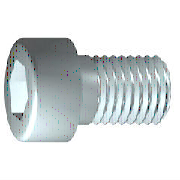
# Autodesk Inventor part: BS EN ISO 4762 - M3 x 10
Saved by Autodesk Inventor 2025.1 (Build 291241000, 241)
## iProperties
Created: 2024-01-20
Part Number: BS EN ISO 4762 - M3 x 10
Material: Acier, doux
Description: Vis cylindrique à six pans creux
Document SubType Name: Modeling
Standard: BS EN ISO 4762
Designer: felix
Standard Revision: 2004
Standards Organization: BSI
Language: fr-FR
Size Designation: M3 x 10
Categories: <MemberInstance><Categories><Category DisplayName="Visserie" InternalName="e4da775c-781d-43d5-af7c-5136215cf5a6" Mnemonic="FSTN"><Category DisplayName="Vis" InternalName="536e6df0-f778-49ac-b2f2-25c71d2aa0b2" Mnemonic="SCRW"><CategoryParameter DisplayName="Désignation du diamètre nominal" InternalName="03caf894-eafd-4c09-a035-916ac084b87b" Mnemonic="nomdiadesig"/><CategoryParameter DisplayName="Longueur nominale" InternalName="238ecbaf-3e6c-45dd-aa95-4068c8e0fd02" Mnemonic="nomlen"/><CategoryParameter DisplayName="Désignation du filetage" InternalName="586d5e89-370a-4089-914f-0110033585c7" Mnemonic="thrdesign"/><CategoryParameter DisplayName="Désignation de série de filetage" InternalName="87c5849c-b3a5-4c3e-9c9b-2feecef9be86" Mnemonic="thrserdsgn"/><CategoryParameter DisplayName="Diamètre nominal" InternalName="8bbe3f8e-44cf-40a9-a251-3a6edc8168d6" Mnemonic="nomdia"/><CategoryParameter DisplayName="Type de taraudage" InternalName="b4bbb7bc-d6aa-4c9f-a9a9-4152b9f6fe49" Mnemonic="thrtype"/><CategoryParameter DisplayName="Pas de filetage" InternalName="bb82302e-82d8-4176-8fc1-c5d7bb17d5ad" Mnemonic="pitch1"/><CategoryParameter DisplayName="Filets par unité" InternalName="bdc6e7d2-ffd0-4d9c-a173-16b95ebb912d" Mnemonic="thrperunit1"/><CategoryParameter DisplayName="Classe de filetage" InternalName="ebc0d23b-2cc6-4d2a-b376-d52aae53bab6" Mnemonic="thrclss"/><Category DisplayName="Tête creuse" InternalName="55e06bf3-7e58-486c-bbdc-745fcc60664d" Mnemonic="CLSCRW"><CategoryParameter DisplayName="Diamètre de tige" InternalName="179dbae3-102f-48bb-85fe-1e3ecd34f7cc" Mnemonic="grpdia"/><CategoryParameter DisplayName="Longueur de filetage" InternalName="3268731d-5f9a-4750-8b01-4a959c46fbf2" Mnemonic="thrlen"/><CategoryParameter DisplayName="Diamètre de tête" InternalName="46177176-dbdd-4a1b-aefd-4c60c45016af" Mnemonic="headdia"/><CategoryParameter DisplayName="Longueur de serrage" InternalName="52eab69f-422f-4795-9995-175a1b827e67" Mnemonic="grplen"/><CategoryParameter DisplayName="Type" InternalName="59a7e495-7a0c-4a5c-bdfd-c090c5f6e2db" Mnemonic="type"/><CategoryParameter DisplayName="Hauteur de tête" InternalName="99c92c4c-4a02-4ebe-9e64-948fb169e19e" Mnemonic="headh"/></Category></Category></Category><Category DisplayName="Type de données" InternalName="23b78d0f-2648-40c6-8793-ca6db495c9e8" Mnemonic="DATATYPE"><CategoryParameter DisplayName="AfficherNom" InternalName="05415f3d-3907-474b-a020-eb9d644f4cf3" Mnemonic="DISPLAYNAME"/><CategoryParameter DisplayName="Norme" InternalName="0c0a119c-1e12-4c84-803f-101930972f5e" Mnemonic="STANDARD"/><CategoryParameter DisplayName="Description" InternalName="13903e3d-64b1-4950-80da-f627842ea37f" Mnemonic="DESCRIPTION"/><CategoryParameter DisplayName="Désignation" InternalName="2675968c-4ce5-49e0-a4f5-552d29089031" Mnemonic="DESIGNATION"/><CategoryParameter DisplayName="Ligne par défaut" InternalName="2af9ec52-faaa-4026-b378-f9fa4afca842" Mnemonic="DEFAULTROW"/><CategoryParameter DisplayName="Nom de dossier" InternalName="3f06958e-8713-4116-9be7-ed6184ecc97b" Mnemonic="FOLDERNAME"/><CategoryParameter DisplayName="Guide révision" InternalName="45a75005-10b1-4dfc-8d6d-dfe629f0b93c" Mnemonic="REVISIONGUID"/><CategoryParameter DisplayName="NomFichier" InternalName="8b46a4cc-9585-4fed-90c3-899f57e09a73" Mnemonic="FILENAME"/><CategoryParameter DisplayName="OrgNorm" InternalName="8f5914e1-4693-403f-8ab5-d37768198c9d" Mnemonic="STDSORG"/><CategoryParameter DisplayName="Version de la famille" InternalName="914462f6-6e19-4b14-ba84-155b9680b1d0" Mnemonic="FAMILYREVISION"/><CategoryParameter DisplayName="Version standard" InternalName="91d5a463-65c2-4fde-b823-3b7fea5e8e17" Mnemonic="STANDARDREVISION"/><CategoryParameter DisplayName="Révision de membre" InternalName="a65d44b9-392f-4f4f-857b-e4b3d54996fe" Mnemonic="MEMBERREVISION"/><CategoryParameter DisplayName="DélimiterFormat" InternalName="bc51e27b-3422-4e78-93ef-cec197ddf230" Mnemonic="CLIPFORMAT"/><CategoryParameter DisplayName="Fabricant" InternalName="cd6c7a72-a28a-4e50-99a9-2c7f4e13e5ad" Mnemonic="MANUFACTURER"/><CategoryParameter DisplayName="NomInterne" InternalName="cf1d0246-76d9-4b4a-8305-fa0409afb5c1" Mnemonic="INTERNALNAME"/><CategoryParameter DisplayName="Métrique" InternalName="e2385c5b-1ea4-4823-96a8-8de651266ec3" Mnemonic="ISMETRIC"/><Category DisplayName="Pièce" InternalName="c0e0b642-3bcb-4cc8-9e80-f96d35c4afa4" Mnemonic="PART"><CategoryParameter DisplayName="Numéro de pièce" InternalName="016b6077-bfbe-49bd-92c9-d8d59c39c941" Mnemonic="PARTNUMBER"/><CategoryParameter DisplayName="Numéro de stock" InternalName="4dba7c1c-e26c-444e-836c-b08b433409a8" Mnemonic="STOCKNUMBER"/><CategoryParameter DisplayName="Clé matière" InternalName="5c9a8adb-dd2b-4535-b97f-0a94a95fe41f" Mnemonic="MATERIALKEY"/><CategoryParameter DisplayName="Matière" InternalName="818a152a-d3c3-49ca-80ee-df7d91421b8e" Mnemonic="MATERIAL"/></Category></Category><Category DisplayName="CarteHéritée" InternalName="cd87c42b-3e48-431e-b5c0-1cbeb14dfe77" Mnemonic="LEGACYMAP"><CategoryParameter DisplayName="ID membre DA unique" InternalName="0918ad47-427f-4fed-ae26-24c81c58f590" Mnemonic="DACOOKIE"/><CategoryParameter DisplayName="ID de fusion11" InternalName="0ee8fb18-e2ed-4f39-96f6-1f4b5f50aa71" Mnemonic="MERGE11"/><CategoryParameter DisplayName="ID membre CC unique" InternalName="5193edd4-b2b0-4ab4-9d54-de900eee34e0" Mnemonic="CCCOOKIE"/><CategoryParameter DisplayName="ID de division" InternalName="72b5c83c-be7f-45c4-ae51-9160ea6deb26" Mnemonic="SPLIT"/><CategoryParameter DisplayName="IDMembre" InternalName="8e5e0294-fc51-4c8f-b3d7-003dc5ed94f6" Mnemonic="MEMBERID"/><CategoryParameter DisplayName="NomCatologue" InternalName="d99d1e27-aa94-4de2-af4c-c348882a6f4f" Mnemonic="CATALOGNAME"/><CategoryParameter DisplayName="NuméroFamille" InternalName="e705e1f4-09cb-413e-91f9-551b4188271e" Mnemonic="FAMILYNUMBER"/></Category></Categories><FamilyTemplate Id="si0145"><FamilyTemplateParameters><FamilyTemplateParameter ObjectType="kUserParameterObject" ValueType="xs:double" Id="1" ObjectReferenceKey="GUL"/><FamilyTemplateParameter ObjectType="kUserParameterObject" ValueType="xs:double" Id="2" ObjectReferenceKey="SPD"/><FamilyTemplateParameter ObjectType="kUserParameterObject" ValueType="xs:double" Id="3" ObjectReferenceKey="NLG"/><FamilyTemplateParameter ObjectType="kUserParameterObject" ValueType="xs:double" Id="4" ObjectReferenceKey="KOD"/><FamilyTemplateParameter ObjectType="kUserParameterObject" ValueType="xs:double" Id="5" ObjectReferenceKey="TOA"/><FamilyTemplateParameter ObjectType="kUserParameterObject" ValueType="xs:double" Id="6" ObjectReferenceKey="GD1"/><FamilyTemplateParameter ObjectType="kUserParameterObject" ValueType="xs:double" Id="7" ObjectReferenceKey="GEL"/><FamilyTemplateParameter ObjectType="kUserParameterObject" ValueType="xs:double" Id="8" ObjectReferenceKey="SW"/><FamilyTemplateParameter ObjectType="kUserParameterObject" ValueType="xs:double" Id="9" ObjectReferenceKey="THREADDIA"/><FamilyTemplateParameter ObjectType="kUserParameterObject" ValueType="xs:double" Id="10" ObjectReferenceKey="INTI"/><FamilyTemplateParameter ObjectType="kUserParameterObject" ValueType="xs:double" Id="11" ObjectReferenceKey="BDM"/><FamilyTemplateParameter ObjectType="kUserParameterObject" ValueType="xs:double" Id="12" ObjectReferenceKey="FAWI"/><FamilyTemplateParameter ObjectType="kUserParameterObject" ValueType="xs:double" Id="13" ObjectReferenceKey="RR"/><FamilyTemplateParameter ObjectType="kUserParameterObject" ValueType="xs:double" Id="14" ObjectReferenceKey="KOH"/><FamilyTemplateParameter ObjectType="kUserParameterObject" ValueType="xs:double" Id="15" ObjectReferenceKey="TPU"/><FamilyTemplateParameter ObjectType="kUserParameterObject" ValueType="xs:double" Id="16" ObjectReferenceKey="PTC"/><FamilyTemplateParameter ObjectType="kUserParameterObject" ValueType="xs:double" Id="17" ObjectReferenceKey="NND"/><FamilyTemplateParameter ObjectType="kUserParameterObject" ValueType="xs:double" Id="18" ObjectReferenceKey="GD"/><FamilyTemplateParameter ObjectType="kUserParameterObject" ValueType="xs:double" Id="19" ObjectReferenceKey="GAL"/><FamilyTemplateParameter ObjectType="kUserParameterObject" ValueType="xs:double" Id="20" ObjectReferenceKey="E0"/><FamilyTemplateParameter ObjectType="kPropertyObject" ValueType="xs:string" Id="100" ObjectReferenceKey="{32853F0F-3444-11d1-9E93-0060B03C1CA6}" SubObjectId="52"/><FamilyTemplateParameter ObjectType="kPropertyObject" ValueType="xs:string" Id="105" ObjectReferenceKey="{32853F0F-3444-11d1-9E93-0060B03C1CA6}" SubObjectId="5"/><FamilyTemplateParameter ObjectType="kPartComponentDefinitionObject" ValueType="xs:string" Id="110" SubObjectId="Material"/><FamilyTemplateParameter ObjectType="kThreadFeatureObject" ValueType="xs:structure" Id="300" ObjectReferenceKey="1002000010000000a2070000000000008000000000000000" SubObjectId="ThreadInfo"><FamilyTemplateParameter ObjectType="" ValueType="xs:string" Id="301" SubObjectId="ThreadDesignation"/><FamilyTemplateParameter ObjectType="" ValueType="xs:string" Id="302" SubObjectId="ThreadType"/><FamilyTemplateParameter ObjectType="" ValueType="xs:string" Id="303" SubObjectId="ThreadClass"/></FamilyTemplateParameter></FamilyTemplateParameters></FamilyTemplate><CategoryParameterMap><ParamToTemplateMap><ParamToTemplate CategoryParameter="//CategoryParameter[@InternalName='05415f3d-3907-474b-a020-eb9d644f4cf3']" ConstantValue="BS EN ISO 4762 - Metric"/><ParamToTemplate CategoryParameter="//CategoryParameter[@InternalName='cf1d0246-76d9-4b4a-8305-fa0409afb5c1']" ConstantValue="7fb936da-4729-46d8-883f-4a5e02d33689"/><ParamToTemplate CategoryParameter="//CategoryParameter[@InternalName='3f06958e-8713-4116-9be7-ed6184ecc97b']" ConstantValue="BS EN ISO 4762"/><ParamToTemplate CategoryParameter="//CategoryParameter[@InternalName='914462f6-6e19-4b14-ba84-155b9680b1d0']" ConstantValue="10"/><ParamToTemplate CategoryParameter="//CategoryParameter[@InternalName='bc51e27b-3422-4e78-93ef-cec197ddf230']" ConstantValue="CF_INVENTOR.STDPARTS"/><ParamToTemplate CategoryParameter="//CategoryParameter[@InternalName='e2385c5b-1ea4-4823-96a8-8de651266ec3']" ConstantValue="true"/><ParamToTemplate CategoryParameter="//CategoryParameter[@InternalName='13903e3d-64b1-4950-80da-f627842ea37f']" ConstantValue="Hexagon Socket Head Cap Screw"/><ParamToTemplate CategoryParameter="//CategoryParameter[@InternalName='8f5914e1-4693-403f-8ab5-d37768198c9d']" ConstantValue="BSI"/><ParamToTemplate CategoryParameter="//CategoryParameter[@InternalName='0c0a119c-1e12-4c84-803f-101930972f5e']" ConstantValue="BS EN ISO 4762"/><ParamToTemplate CategoryParameter="//CategoryParameter[@InternalName='cd6c7a72-a28a-4e50-99a9-2c7f4e13e5ad']" TemplateParameter="104"/><ParamToTemplate CategoryParameter="//CategoryParameter[@InternalName='91d5a463-65c2-4fde-b823-3b7fea5e8e17']" ConstantValue="2004"/><ParamToTemplate CategoryParameter="//CategoryParameter[@InternalName='45a75005-10b1-4dfc-8d6d-dfe629f0b93c']" ConstantValue="41658f13-6969-4cd7-b79b-4322ed6d28fd"/><ParamToTemplate CategoryParameter="//CategoryParameter[@InternalName='2af9ec52-faaa-4026-b378-f9fa4afca842']" ConstantValue="10"/><ParamToTemplate CategoryParameter="//CategoryParameter[@InternalName='d99d1e27-aa94-4de2-af4c-c348882a6f4f']" ConstantValue="BSI"/><ParamToTemplate CategoryParameter="//CategoryParameter[@InternalName='e705e1f4-09cb-413e-91f9-551b4188271e']" ConstantValue="12"/><ParamToTemplate CategoryParameter="//CategoryParameter[@InternalName='8b46a4cc-9585-4fed-90c3-899f57e09a73']" ConstantValue="BS EN ISO 4762 - M3 x 10(1)"/><ParamToTemplate CategoryParameter="//CategoryParameter[@InternalName='a65d44b9-392f-4f4f-857b-e4b3d54996fe']" ConstantValue="96AC4FB5-6517-466C-9B8C-79DF0343AFBC"/><ParamToTemplate CategoryParameter="//CategoryParameter[@InternalName='52eab69f-422f-4795-9995-175a1b827e67']" ConstantValue="1,25"/><ParamToTemplate CategoryParameter="//CategoryParameter[@InternalName='ebc0d23b-2cc6-4d2a-b376-d52aae53bab6']" ConstantValue="6g"/><ParamToTemplate CategoryParameter="//CategoryParameter[@InternalName='03caf894-eafd-4c09-a035-916ac084b87b']" ConstantValue="M3"/><ParamToTemplate CategoryParameter="//CategoryParameter[@InternalName='b4bbb7bc-d6aa-4c9f-a9a9-4152b9f6fe49']" ConstantValue="ISO Metric profile"/><ParamToTemplate CategoryParameter="//CategoryParameter[@InternalName='8e5e0294-fc51-4c8f-b3d7-003dc5ed94f6']" ConstantValue="310"/><ParamToTemplate CategoryParameter="//CategoryParameter[@InternalName='179dbae3-102f-48bb-85fe-1e3ecd34f7cc']" TemplateParameter="11"/><ParamToTemplate CategoryParameter="//CategoryParameter[@InternalName='2675968c-4ce5-49e0-a4f5-552d29089031']" TemplateParameter="100"/><ParamToTemplate CategoryParameter="//CategoryParameter[@InternalName='3268731d-5f9a-4750-8b01-4a959c46fbf2']" TemplateParameter="7"/><ParamToTemplate CategoryParameter="//CategoryParameter[@InternalName='46177176-dbdd-4a1b-aefd-4c60c45016af']" TemplateParameter="4"/><ParamToTemplate CategoryParameter="//CategoryParameter[@InternalName='99c92c4c-4a02-4ebe-9e64-948fb169e19e']" TemplateParameter="14"/><ParamToTemplate CategoryParameter="//CategoryParameter[@InternalName='818a152a-d3c3-49ca-80ee-df7d91421b8e']" TemplateParameter="110"/><ParamToTemplate CategoryParameter="//CategoryParameter[@InternalName='238ecbaf-3e6c-45dd-aa95-4068c8e0fd02']" TemplateParameter="3"/><ParamToTemplate CategoryParameter="//CategoryParameter[@InternalName='8bbe3f8e-44cf-40a9-a251-3a6edc8168d6']" TemplateParameter="17"/><ParamToTemplate CategoryParameter="//CategoryParameter[@InternalName='016b6077-bfbe-49bd-92c9-d8d59c39c941']" TemplateParameter="105"/><ParamToTemplate CategoryParameter="//CategoryParameter[@InternalName='bb82302e-82d8-4176-8fc1-c5d7bb17d5ad']" TemplateParameter="16"/><ParamToTemplate CategoryParameter="//CategoryParameter[@InternalName='586d5e89-370a-4089-914f-0110033585c7']" TemplateParameter="301"/><ParamToTemplate CategoryParameter="//CategoryParameter[@InternalName='bdc6e7d2-ffd0-4d9c-a173-16b95ebb912d']" TemplateParameter="15"/></ParamToTemplateMap></CategoryParameterMap></MemberInstance>
Density: 7.85 g/cm^3
Appearance: Semi-poli
IsCustomPart: 0
Author: felix
Autodesk Inventor part; units mm, degrees
ref_plane "YZ Plane" through (0, 0, 0) normal (1, 0, 0) x (0, 1, 0)
ref_plane "XZ Plane" through (0, 0, 0) normal (0, 1, 0) x (-1, 0, 0)
sketch "Esquisse1" plane through (0, 0, 0) normal (0, 0, 1) x (1, 0, 0)
  line L0 (-0.8667, 0) -> (10, 0)
  line L1 (10, 0) -> (10, 1.5)
  line L2 (10, 1.5) -> (1.25, 1.5)
  line L3 (1.25, 1.5) -> (0.9432, 1.5)
  line L4 (0.9432, 1.5) -> (0, 1.5)
  line L5 (0, 1.5) -> (0, 2.75)
  line L6 (0, 2.75) -> (-3, 2.75)
  line L7 (-3, 2.75) -> (-3, 1.4434)
  line L8 (-3, 1.4434) -> (-1.7, 1.4434)
  line L9 (-1.7, 1.4434) -> (-0.8667, 0)
  line L10 (-5.6, 0) -> (12.6, 0) projected
  line L11 (0, -0.55) -> (0, 3.3) projected
  line L12 (1.25, 1.5) -> (0, 1.5) construction
  dimension "d1" = 8.75
  dimension "d2" = 0.3068
  dimension "d3" = 3
  dimension "d4" = 1.3
  dimension "d5" = 60
  dimension "d6" = 3
  dimension "d7" = 3
  dimension "d8" = 2.8868
  dimension "d9" = 5.5
  dimension "d26" = 10
  constraints: 22 end point, 6 parallel, 2 collinear, 2 perpendicular, 1 horizontal, 1 point on line
  measures "d1" distance from line of L2.end L1
  measures "d2" distance of L3.end L2.end
  measures "d3" distance between parallel lines of L7 L5
  measures "d4" distance of L7.end L8.end
  measures "d5" angle of L9 L0
  measures "d6" diameter of L2 L0
  measures "d7" diameter of L4 L0
  measures "d8" diameter of L8 L0
  measures "d9" diameter of L6 L0
  measures "d26" distance between parallel lines of L11 L1
revolve "Corps" add sketch "Esquisse1" angle 360 about axis through (-0.8667, 0, 0) along (1, 0, 0)
sketch "Esquisse2" plane through (-3, 0, 0) normal (-1, 0, 0) x (0, 0, 1)
  circle A0 centre (0, 0) radius 1.4434 projected
  line L0 (0, -3.85) -> (0, 3.85) projected
  line L1 (-3.85, 0) -> (3.85, 0) projected
  line L2 (1.4434, 0) -> (0.7217, -1.25)
  line L3 (0.7217, -1.25) -> (-0.7217, -1.25)
  line L4 (-0.7217, -1.25) -> (-1.4434, 0)
  line L5 (-1.4434, 0) -> (-0.7217, 1.25)
  line L6 (-0.7217, 1.25) -> (0.7217, 1.25)
  line L7 (0.7217, 1.25) -> (1.4434, 0)
  point P0 (0, 0)
  constraints: 12 end point, 1 coincident, 1 horizontal alignment, 1 point on line, 12 other
extrude "Rainure" add sketch "Esquisse2" against normal up to next contours L7 A0 | A0 L2 | L6 L0 A0 | A0 L0 L3 | L0 L6 A0 | A0 L3 L0 | L4 A0 | A0 L5
fillet "Congé1" radius 0.3 1 edges at (-3, -2.75, 0)
thread "Filetage" size "M3x0.5" class "6g" standard "ISO Metric profile" length 8.75
chamfer "Chanfrein1" distance 0.3067 distance2 0.3067 1 edges at (10, -1.5, 0) measured on face at (10, -1, 0)
ref_plane "Work Plane1" through (29, 0, 0) normal (0, -1, 0) x (1, 0, 0)
fillet "Fillet2" radius 0.1 1 edges at (0, -1.5, 0)
equation "\"d30\" = R"
equation "\"d17\" = RR"
equation "\"d13\" = GEL"
equation "\"d15\" = -0.5 * SPD + 0.5 * GD"
equation "\"d16\" = GUL"
equation "\"d1\" = GEL"
equation "\"d3\" = KOH"
equation "\"d4\" = INTI"
equation "\"d6\" = GD"
equation "\"d7\" = BDM"
equation "\"d8\" = 1.1547 * SW"
equation "\"d9\" = KOD"
equation "\"d26\" = NLG"
equation "\"GD\" = NND"
equation "\"NLG\" = 10"
equation "\"GEL\" = 8.75"
equation "\"KOD\" = 5.5"
equation "\"KOH\" = NND"
equation "\"INTI\" = 1.3"
equation "\"GAL\" = 0.61345 * PTC"
equation "\"GUL\" = 0.61345 * PTC"
equation "\"BDM\" = NND"
equation "\"SW\" = 2.5"
equation "\"RR\" = 0.1 * NND"
equation "\"SPD\" = NND - 1.2269 * PTC"
equation "\"R\" = 0.1"
equation "\"TOA\" = 30deg"
equation "\"GD1\" = THREADDIA - 1.2269 * PTC"
equation "\"THREADDIA\" = NND"
equation "\"FAWI\" = 45deg"
equation "\"PTC\" = 0.5"
equation "\"NND\" = 3"
equation "\"E0\" = 1.155 * SW"
body "Solid1"
